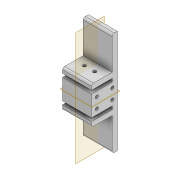
# Autodesk Inventor part: Foam_wing_mount
Saved by Autodesk Inventor 2022 (Build 260153000, 153)
## iProperties
Created: 2022-06-29
Part Number: Foam_wing_mount
Material: Generic
Document SubType Name: Modeling
Designer: dell
Density: 1 g/cm^3
Appearance: Default
Mass: 30.3471 g
Surface Area: 119.338 cm^2
Volume: 30.3471 cm^3
Author: dell
Autodesk Inventor part; units mm, degrees
ref_plane "YZ Plane" through (0, 0, 0) normal (1, 0, 0) x (0, 1, 0)
ref_plane "XZ Plane" through (0, 0, 0) normal (0, 1, 0) x (-1, 0, 0)
ref_plane "XY Plane" through (0, 0, 0) normal (0, 0, 1) x (1, 0, 0)
sketch "Sketch1" plane through (0, 0, 0) normal (0, 0, 1) x (1, 0, 0)
  line L0 (0, 0) -> (28, 0)
  line L1 (28, 0) -> (28, 100)
  line L2 (28, 100) -> (0, 100)
  line L3 (0, 100) -> (0, 0)
  dimension "d0" = 28
  dimension "d1" = 100
  constraints: 8 end point, 2 parallel, 1 horizontal, 1 perpendicular
  measures "d0" distance between parallel lines of L3 L1
  measures "d1" distance between parallel lines of L0 L2
extrude "Extrusion1" add sketch "Sketch1" along normal blind 5
sketch "Sketch3" plane through (0, 0, 5) normal (0, 0, 1) x (1, 0, 0)
  line L0 (28, 0) -> (28, 100) projected
  line L1 (28, 100) -> (0, 100) projected
  line L2 (0, 100) -> (0, 0) projected
  line L3 (0, 0) -> (28, 0) projected
  line L4 (0, 50) -> (28, 50) construction
  line L5 (28, 0) -> (28, 100) construction
  line L6 (0, 100) -> (0, 0) projected
  line L7 (0, 60) -> (28, 60)
  line L8 (28, 60) -> (28, 40)
  line L9 (28, 40) -> (0, 40)
  line L10 (0, 40) -> (0, 60)
  line L11 (0, 63.1) -> (28, 63.1)
  line L12 (28, 63.1) -> (28, 68.1)
  line L13 (28, 68.1) -> (0, 68.1)
  line L14 (0, 68.1) -> (0, 63.1)
  line L15 (0, 36.9) -> (28, 36.9)
  line L16 (28, 36.9) -> (28, 31.9)
  line L17 (28, 31.9) -> (0, 31.9)
  line L18 (0, 31.9) -> (0, 36.9)
  point P0 (0, 31.9)
  point P1 (28, 36.9)
  point P2 (0, 40)
  point P3 (0, 68.1)
  point P4 (28, 63.1)
  dimension "d6" = 50
  dimension "d7" = 100
  dimension "d8" = 10
  dimension "d9" = 10
  dimension "d10" = 5
  dimension "d11" = 3.1
  dimension "d12" = 3.1
  dimension "d13" = 5
  constraints: 26 end point, 6 parallel, 6 point on line, 4 perpendicular, 3 horizontal, 2 midpoint
  measures "d6" distance between parallel lines of L3 L4
  measures "d7" distance between parallel lines of L1 L3
  measures "d8" distance between parallel lines of L4 L9
  measures "d9" distance between parallel lines of L4 L7
  measures "d10" distance between parallel lines of L13 L11
  measures "d11" distance between parallel lines of L7 L11
  measures "d12" distance between parallel lines of L9 L15
  measures "d13" distance between parallel lines of L17 L15
extrude "Extrusion2" add sketch "Sketch3" along normal blind 20 contours L17 L2 L15 L0 | L9 L2 L7 L0 | L11 L2 L13 L0
sketch "Sketch4" plane through (0, 68.1, 5) normal (0, 1, 0) x (1, 0, 0)
  line L0 (0, 0) -> (28, 0) projected
  line L1 (0, 0) -> (0, -20) projected
  line L2 (28, -20) -> (0, -20) projected
  line L3 (28, 0) -> (28, -20) projected
  circle A0 centre (9.05, -8) radius 1.55
  circle A1 centre (18.95, -8) radius 1.55
  line L4 (0, -20) -> (28, -20) construction
  line L5 (14, -20) -> (14, 0) construction
  point P0 (0, 5)
  dimension "d16" = 3.1
  dimension "d17" = 3.1
  dimension "d18" = 4.95
  dimension "d19" = 4.95
  dimension "d20" = 8
  dimension "d21" = 8
  constraints: 2 centre point, 2 end point, 2 midpoint
  measures "d16" diameter of A0
  measures "d17" diameter of A1
  measures "d18" distance from line of L5 A0.centre
  measures "d19" distance from line of A1.centre L5
  measures "d20" distance from line of L0 A1.centre
  measures "d21" distance from line of L0 A0.centre
extrude "Extrusion3" cut sketch "Sketch4" against normal blind 100 contours A0 | A1
ref_plane "Work Plane1" through (14, 0, 0) normal (1, 0, 0) x (0, 0, -1)
sketch "Sketch13" plane through (28, 0, 0) normal (1, 0, 0) x (0, 0, -1)
  circle A0 centre (-5, 55) radius 1.5
  circle A1 centre (-5, 45) radius 1.5
  circle A2 centre (-20, 55) radius 1.5
  circle A3 centre (-20, 45) radius 1.5
  line L0 (-5, 60) -> (-25, 60) projected
  line L1 (-5, 40) -> (-25, 40) projected
  line L2 (-25, 40) -> (-25, 60) projected
  line L3 (0, 0) -> (0, 100) projected
  dimension "d57" = 3
  dimension "d58" = 3
  dimension "d59" = 3
  dimension "d60" = 3
  dimension "d61" = 5
  dimension "d62" = 5
  dimension "d63" = 5
  dimension "d64" = 5
  dimension "d65" = 5
  dimension "d67" = 5
  dimension "d69" = 5
  dimension "d70" = 5
  constraints: 4 centre point
  measures "d57" diameter of A0
  measures "d58" diameter of A1
  measures "d59" diameter of A2
  measures "d60" diameter of A3
  measures "d61" distance from line of L0 A0.centre
  measures "d62" distance from line of L0 A2.centre
  measures "d63" distance from line of L1 A1.centre
  measures "d64" distance from line of L1 A3.centre
  measures "d65" distance from line of L2 A3.centre
  measures "d67" distance from line of A2.centre L2
  measures "d69" distance from line of L3 A1.centre
  measures "d70" distance from line of L3 A0.centre
extrude "Extrusion11" cut sketch "Sketch13" against normal blind 180
fillet "Fillet1" radius 2 4 edges at (14, 100, 5) (14, 0, 5) (14, 68.1, 25) (14, 31.9, 25)
ref_plane "Work Plane3" through (0, 50, 5) normal (0, 1, 0) x (1, 0, 0)
equation "\"d6\" = 0.5 * d7"
equation "\"d62\" = d61"
equation "\"d63\" = d61"
equation "\"d64\" = d61"
equation "\"d67\" = d65"
equation "\"d69\" = d65"
equation "\"d70\" = d65"
body "Solid1"
